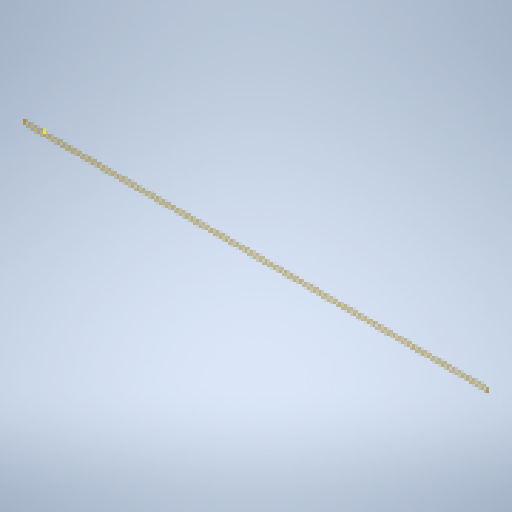
# Autodesk Inventor part: низочек
Saved by Autodesk Inventor 2024.2 (Build 282272000, 272)
## iProperties
Created: 2025-11-21
Part Number: низочек
Material: Типовые
Document SubType Name: Modeling
Designer: Zakhar
Density: 1 g/cm^3
Appearance: По умолчанию
Author: Zakhar
Autodesk Inventor part; units mm, degrees
ref_plane "YZ Plane" through (0, 0, 0) normal (1, 0, 0) x (0, 1, 0)
ref_plane "XZ Plane" through (0, 0, 0) normal (0, 1, 0) x (-1, 0, 0)
ref_plane "XY Plane" through (0, 0, 0) normal (0, 0, 1) x (1, 0, 0)
ref_plane "РабПлоскость1" through (0, 0, 0) normal (0, 0, 1) x (1, 0, 0)
sketch "Эскиз1" plane through (0, 0, 0) normal (0, 0, 1) x (1, 0, 0)
  line L0 (0, 0) -> (2010.3464, 0)
  line L1 (2010.3464, 0) -> (2010.3464, -242.7293)
  line L2 (2010.3464, -242.7293) -> (0, -242.7293)
  line L3 (0, -242.7293) -> (0, 0)
  constraints: 8 end point, 2 parallel, 1 horizontal, 1 perpendicular
extrude "Выдавливание1" add sketch "Эскиз1" along normal blind 10
